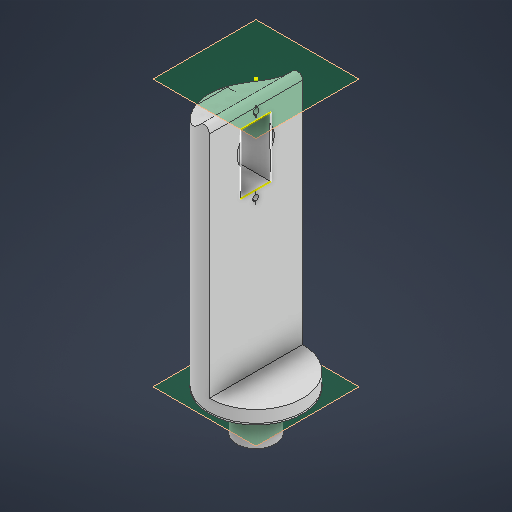
# Autodesk Inventor part: p1
Saved by Autodesk Inventor 2026.2 (Build 302298000, 298)
## iProperties
Created: 2026-03-23
Part Number: p1
Material: Generic
Document SubType Name: Modeling
Designer: anasa
Density: 1 g/cm^3
Appearance: Default
Author: anasa
Autodesk Inventor part; units mm, degrees
ref_plane "XZ Plane" through (0, 0, 0) normal (0, 1, 0) x (-1, 0, 0)
sketch "Sketch1" plane through (0, 0, 0) normal (0, 1, 0) x (-1, 0, 0)
  circle A0 centre (0, 0) radius 50
  line L0 (0, 0) -> (0, -94.0915) construction
  circle A1 centre (0, 0) radius 35 construction
  circle A2 centre (0, -35) radius 5
  circle A3 centre (35, 0) radius 5
  circle A4 centre (0, 35) radius 5
  circle A5 centre (-35, 0) radius 5
  dimension "d1" = 70
  dimension "d0" = 100
  dimension "d2" = 10
  dimension "d5" = 360
  constraints: 5 centre point, 2 coincident, 2 end point, 1 point on line, 1 vertical, 1 vertical alignment, 11 other
  measures "d0" diameter of A0
  measures "d2" diameter of A2
extrude "Extrusion1" add sketch "Sketch1" along normal blind 3.5
sketch "Sketch2" plane through (0, 3.5, 0) normal (0, 1, 0) x (1, 0, 0)
  circle A0 centre (0, 0) radius 17.5
  dimension "d9" = 35
  constraints: 1 centre point, 1 coincident
  measures "d9" diameter of A0
extrude "Extrusion2" add sketch "Sketch2" along normal blind 100
ref_plane "Work Plane1" through (0, 0, 0) normal (1, 0, 0) x (0, 1, 0)
sketch "Sketch3" plane through (0, 0, 0) normal (1, 0, 0) x (0, 1, 0)
  point P0 (0, 0)
sketch "Sketch4" plane through (0, 0, 0) normal (1, 0, 0) x (0, 1, 0)
  line L0 (68.9724, 5.8) -> (91.4724, 5.8)
  line L1 (91.4724, 5.8) -> (91.4724, -5.5)
  line L2 (91.4724, -5.5) -> (68.9724, -5.5)
  line L3 (68.9724, -5.5) -> (68.9724, 5.8)
  line L4 (68.9724, 5.8) -> (91.4724, -5.5) construction
  line L5 (91.4724, 5.8) -> (68.9724, -5.5) construction
  point P0 (0, 0)
  point P1 (80.2224, 0.15)
  dimension "d13" = 22.5
  dimension "d14" = 11.3
  constraints: 12 end point, 2 midpoint, 2 parallel, 1 horizontal, 1 perpendicular
  measures "d13" distance of L1.end L2.end
  measures "d14" distance of L0.end L1.end
extrude "Extrusion3" cut sketch "Sketch4" against normal blind 100
sketch "Sketch5" plane through (0, 0, 0) normal (1, 0, 0) x (0, 1, 0)
  line L0 (91.4724, -5.5) -> (91.4724, 5.8) projected
  line L1 (68.9724, 5.8) -> (68.9724, -5.5) projected
  line L2 (91.4724, -5.5) -> (68.9724, -5.5)
  line L3 (68.9724, -5.5) -> (68.9724, 5.8)
  line L4 (68.9724, 5.8) -> (91.4724, 5.8)
  line L5 (91.4724, 5.8) -> (91.4724, -5.5)
  point P0 (0, 0)
  constraints: 8 end point, 2 parallel, 1 horizontal, 1 perpendicular
sketch "Sketch6" plane through (0, 103.5, 0) normal (0, 1, 0) x (1, 0, 0)
  circle A0 centre (0, 0) radius 17.5
  line L0 (0, 17.5) -> (0, -17.5)
  dimension "d17" = 35
  dimension "d18" = 35
  constraints: 2 end point, 2 point on circle, 1 centre point, 1 coincident, 1 vertical
  measures "d17" diameter of A0
  measures "d18" distance of L0.start L0.end
extrude "Extrusion4" cut sketch "Sketch6" against normal blind 50 contours A0 L0 picked at (4.9351, 4.4144)
sketch "Sketch7" plane through (0, 103.5, 17.5) normal (1, 0, 0) x (0, 0, -1)
  circle A0 centre (17.5, -9.0276) radius 1.1
  circle A1 centre (17.35, -37.0276) radius 1.1
  line L0 (0, 0) -> (35, 0) projected
  line L1 (11.7, -34.5276) -> (23, -34.5276) projected
  line L2 (23, -12.0276) -> (11.7, -12.0276) projected
  point P0 (17.5, -103.5)
  point P1 (17.5, 0)
  point P2 (17.35, -34.5276)
  dimension "d21" = 2.2
  dimension "d22" = 2.2
  dimension "d23" = 28
  dimension "d24" = 2.5
  dimension "d25" = 3
  constraints: 2 centre point, 2 midpoint, 2 vertical alignment
  measures "d21" diameter of A0
  measures "d22" diameter of A1
  measures "d23" vertical distance of A1.centre A0.centre
  measures "d24" distance from line of L1 A1.centre
  measures "d25" distance from line of L2 A0.centre
extrude "Extrusion5" cut sketch "Sketch7" against normal blind 4
sketch "Sketch8" plane through (0, 103.5, 17.5) normal (1, 0, 0) x (0, 0, -1)
  line L0 (17.2, -39.1295) -> (17.5, -39.1295)
  line L1 (17.5, -39.1295) -> (17.5, -34.9258)
  line L2 (17.5, -34.9258) -> (17.2, -34.9258)
  line L3 (17.2, -34.9258) -> (17.2, -39.1295)
  circle A0 centre (17.35, -37.0276) radius 1.1 projected
  line L4 (17.2, -39.1295) -> (17.5, -34.9258) construction
  line L5 (17.5, -39.1295) -> (17.2, -34.9258) construction
  line L6 (17.65, -11.0326) -> (17.35, -11.0326)
  line L7 (17.35, -11.0326) -> (17.35, -7.0227)
  line L8 (17.35, -7.0227) -> (17.65, -7.0227)
  line L9 (17.65, -7.0227) -> (17.65, -11.0326)
  circle A1 centre (17.5, -9.0276) radius 1.1 projected
  line L10 (17.65, -11.0326) -> (17.35, -7.0227) construction
  line L11 (17.35, -11.0326) -> (17.65, -7.0227) construction
  line L12 (17.2, -36.8668) -> (17.5, -36.8668)
  line L13 (17.35, -8.7838) -> (17.65, -8.7838)
  point P0 (17.5, -103.5)
  constraints: 28 end point, 4 midpoint, 4 parallel, 4 perpendicular, 4 point on line, 2 horizontal
extrude "Extrusion6" cut sketch "Sketch8" against normal blind 4 contours L3 A0 L1 L0 | L3 L12 L1 A0 | L3 A0 L1 L12 | L3 L2 L1 A0 | L6 L7 A1 L9 | A1 L7 L13 L9 | L13 L7 A1 L9 | L7 L8 L9 A1
ref_plane "Work Plane2" through (0, 0, 0) normal (0, 0, 1) x (1, 0, 0)
sketch "Sketch9" plane through (0, 0, 0) normal (0, 0, 1) x (1, 0, 0)
  line L0 (17.5, 3.5) -> (17.5, 53.5) projected
  line L1 (50, 3.5) -> (-50, 3.5) projected
  line L2 (-17.5, 3.5) -> (-17.5, 103.5) projected
  arc A0 (-17.5, 91.5181) -> (0, 103.5) centre (-16.2539, 108.4688) ccw
  line L3 (0, 91.4724) -> (-16.6132, 91.4724) projected
  line L4 (-17.5, 91.5181) -> (-17.5, 103.5)
  line L5 (-17.5, 91.5181) -> (-17.5, 108.4688)
  line L6 (-17.5, 108.4688) -> (0, 108.4688)
  line L7 (0, 108.4688) -> (0, 103.5)
  line L8 (0, 103.5) -> (0, 53.5) projected
  line L9 (0, 53.5) -> (0, 3.5)
  arc A1 (0, 53.5) -> (17.5, 12.367) centre (50.307, 50.6139) ccw
  line L10 (0, 53.5) -> (17.5, 53.5) projected
  line L11 (0, 53.5) -> (22.4323, 53.5)
  line L12 (22.4323, 53.5) -> (17.5, 12.367)
  point P0 (0, 0)
  point P1 (0, 47.7278)
  constraints: 14 end point, 4 point on circle, 3 perpendicular, 3 point on line, 2 centre point, 1 horizontal, 1 midpoint, 1 tangent
extrude "Extrusion7" cut sketch "Sketch9" along normal through all both and the other way through all contours A1 L9 L10 L0 | L0 L11 L12 | L2 L5 L6 L7 A0
fillet "Fillet1" radius 2 1 edges at (0, 103.5, 0)
fillet "Fillet2" [suppressed]
sketch "Sketch10" plane through (0, 0, 0) normal (0, -1, 0) x (1, 0, 0)
  circle A0 centre (0, -35) radius 5 projected
  circle A1 centre (0, -35) radius 5
  circle A2 centre (-35, 0) radius 5 projected
  circle A3 centre (-35, 0) radius 5
  circle A4 centre (0, 35) radius 5 projected
  circle A5 centre (0, 35) radius 5
  circle A6 centre (35, 0) radius 5 projected
  circle A7 centre (35, 0) radius 5
  point P0 (0, 0)
  constraints: 4 centre point, 4 coincident
extrude "Extrusion8" add sketch "Sketch10" against normal blind 3.5
sketch "Sketch11" plane through (0, 0, 0) normal (0, -1, 0) x (1, 0, 0)
  circle A0 centre (0, 0) radius 17.5 projected
  circle A1 centre (0, 0) radius 45 construction
  line L0 (0, 0) -> (-76.7303, 0) construction
  point P0 (-45, 0)
  point P1 (-22.5, -38.9711)
  point P2 (22.5, -38.9711)
  point P3 (45, 0)
  point P4 (22.5, 38.9711)
  point P5 (-22.5, 38.9711)
  dimension "d39" = 90
  dimension "d42" = 360
  constraints: 2 end point, 1 coincident, 1 horizontal, 1 horizontal alignment, 1 point on line, 9 other
hole "Hole1" at (-45, 0, 0) at (-22.5, 0, -38.9711) at (-22.5, 0, 38.9711) at (22.5, 0, 38.9711) at (45, 0, 0) at (22.5, 0, -38.9711) direction (0, 1, 0) diameter 6.647 depth 22.2 tip angle 118 thread size "M8x1.25" class "6H" standard "ANSI Metric M Profile"
fillet "Fillet3" radius 2 1 edges at (-17.5, 3.5, 0)
sketch "Sketch12" plane through (0, 94.4724, 0) normal (1, 0, 0) x (0, 0, -1)
  circle A0 centre (-0.15, -11) radius 7
  line L0 (5.5, -3) -> (-5.8, -3) projected
  point P0 (0, -94.4724)
  point P1 (-0.15, -3)
  point P2 (-0.15, -3)
  dimension "d52" = 14
  dimension "d53" = 8
  constraints: 2 midpoint, 1 centre point, 1 vertical alignment
  measures "d52" diameter of A0
  measures "d53" distance of A0.centre point (-0.15, -3)
extrude "Extrusion9" cut sketch "Sketch12" against normal blind 0.5
sketch "Sketch13" plane through (0, 0, 0) normal (0, -1, 0) x (1, 0, 0)
  circle A0 centre (0, 0) radius 71.7969
  constraints: 1 centre point, 1 coincident
extrude "Extrusion10" cut sketch "Sketch13" against normal blind 5
sketch "Sketch14" plane through (0, 5, 0) normal (0, -1, 0) x (1, 0, 0)
  circle A0 centre (0, 0) radius 7.25
  dimension "d59" = 14.5
  constraints: 1 centre point, 1 coincident
  measures "d59" diameter of A0
extrude "Extrusion11" add sketch "Sketch14" along normal blind 15
ref_plane "Work Plane3" through (0, 5, 0) normal (0, -1, 0) x (1, 0, 0)
sketch "Sketch15" plane through (0, 5, 0) normal (0, -1, 0) x (1, 0, 0)
  point P0 (0, 0)
ref_plane "Work Plane4" through (0, 105, 0) normal (0, -1, 0) x (1, 0, 0)
sketch "Sketch16" plane through (0, 105, 0) normal (0, -1, 0) x (1, 0, 0)
  point P0 (0, 0)
sketch "Sketch17" plane through (0, 105, 0) normal (0, -1, 0) x (1, 0, 0)
  circle A0 centre (0, 0) radius 27.3383
  line L0 (0, 0) -> (0, 37.7238)
  line L1 (0, 37.7238) -> (0, -33.1122)
  point P0 (0, -27.3383)
  point P1 (0, 27.3383)
  constraints: 4 end point, 1 centre point, 1 coincident, 1 point on line, 1 vertical
extrude "Extrusion12" cut sketch "Sketch17" along normal blind 95 contours A0 L1 L0 picked at (17.9971, -2.0278)
body "Solid1"
